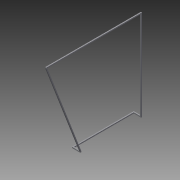
# Autodesk Inventor part: CatchFrameLeft
Saved by Autodesk Inventor 2013 (Build 170138000, 138)
## iProperties
Created: 2014-01-24
Part Number: CatchFrameLeft
Material: Generic
Document SubType Name: Modeling
Designer: Jarod
Density: 1 g/cm^3
Author: Jarod
Autodesk Inventor part; units mm, degrees
ref_plane "YZ Plane" through (0, 0, 0) normal (1, 0, 0) x (0, 1, 0)
ref_plane "XZ Plane" through (0, 0, 0) normal (0, 1, 0) x (-1, 0, 0)
ref_plane "XY Plane" through (0, 0, 0) normal (0, 0, 1) x (1, 0, 0)
sketch "Sketch1" plane through (0, 0, 0) normal (1, 0, 0) x (0, 1, 0)
  line L0 (0, 0) -> (6.35, 0)
  line L1 (6.35, 0) -> (6.35, 381)
  line L2 (6.35, 381) -> (0, 381)
  line L3 (0, 381) -> (0, 0)
  dimension "d0" = 6.35
  dimension "d1" = 381
  constraints: 8 end point, 2 parallel, 1 horizontal, 1 perpendicular
  measures "d0" distance of L2.end L1.end
  measures "d1" distance of L1.end L0.end
extrude "Extrusion1" add sketch "Sketch1" along normal blind 6.35
sketch "Sketch2" plane through (6.35, 0, 0) normal (1, 0, 0) x (0, 0, -1)
  line L0 (-381, 6.35) -> (-374.65, 6.35)
  line L1 (-374.65, 6.35) -> (-374.65, 0)
  line L2 (-374.65, 0) -> (-381, 0)
  line L3 (-381, 0) -> (-381, 6.35)
  line L4 (0, 6.35) -> (-6.35, 6.35)
  line L5 (-6.35, 6.35) -> (-6.35, 0)
  line L6 (-6.35, 0) -> (0, 0)
  line L7 (0, 0) -> (0, 6.35)
  dimension "d4" = 6.35
  dimension "d5" = 6.35
  dimension "d6" = 6.35
  dimension "d7" = 6.35
  constraints: 16 end point, 4 parallel, 2 horizontal, 2 perpendicular
  measures "d4" distance of L1.end L2.end
  measures "d5" distance of L0.end L1.end
  measures "d6" distance of L6.end L5.end
  measures "d7" distance of L5.end L4.end
extrude "Extrusion2" add sketch "Sketch2" along normal blind 38.1
sketch "Sketch3" plane through (44.45, 0, 0) normal (1, 0, 0) x (0, 0, -1)
  line L0 (0, 0) -> (-6.35, 0)
  line L1 (-6.35, 0) -> (-6.35, 558.8)
  line L2 (-6.35, 558.8) -> (0, 558.8)
  line L3 (0, 558.8) -> (0, 0)
  dimension "d10" = 6.35
  dimension "d11" = 558.8
  constraints: 8 end point, 2 parallel, 1 horizontal, 1 perpendicular
  measures "d10" distance of L1.end L2.end
  measures "d11" distance of L0.end L1.end
extrude "Extrusion3" add sketch "Sketch3" along normal blind 6.35
sketch "Sketch4" plane through (50.8, 0, 0) normal (1, 0, 0) x (0, 0, -1)
  line L0 (0, 558.8) -> (-590.55, 558.8)
  line L1 (-590.55, 558.8) -> (-590.55, 552.45)
  line L2 (-590.55, 552.45) -> (0, 552.45)
  line L3 (0, 552.45) -> (0, 558.8)
  dimension "d14" = 590.55
  dimension "d15" = 6.35
  constraints: 8 end point, 2 parallel, 1 horizontal, 1 perpendicular
  measures "d14" distance of L2.end L1.end
  measures "d15" distance of L1.end L0.end
extrude "Extrusion4" add sketch "Sketch4" against normal blind 6.35
sketch "Sketch5" plane through (44.45, 0, 0) normal (1, 0, 0) x (0, 0, -1)
  line L0 (-381, 6.35) -> (-381, 0) projected
  line L1 (-381, 0) -> (-374.65, 0) projected
  line L2 (-374.65, 0) -> (-374.65, 6.35) projected
  line L3 (-374.65, 6.35) -> (-381, 6.35) projected
  line L4 (-381, 6.35) -> (171.45, 6.35) construction
  line L5 (-381, 558.8) -> (-590.55, 558.8)
  line L6 (-590.55, 558.8) -> (-590.55, 552.45)
  line L7 (-590.55, 552.45) -> (-381, 6.35)
  line L8 (-590.55, 558.8) -> (-584.2, 558.8)
  line L9 (-584.2, 558.8) -> (-584.2, 552.45)
  line L10 (-584.2, 552.45) -> (-590.55, 552.45)
  line L11 (-590.55, 552.45) -> (-590.55, 558.8)
  line L12 (-584.2, 552.45) -> (-374.65, 6.35)
  point P0 (0, 0)
  dimension "d18" = 552.45
  dimension "d20" = 209.55
  dimension "d22" = 6.35
  dimension "d23" = 90
  dimension "d24" = 6.35
  dimension "d25" = 6.35
  constraints: 18 end point, 2 horizontal, 2 parallel, 1 perpendicular
  measures "d18" distance of L0.start L5.start
  measures "d20" distance of L5.start L5.end
  measures "d22" distance of L5.end L6.end
  measures "d23" angle of L6 L5
  measures "d24" distance of L9.end L10.end
  measures "d25" distance of L8.end L9.end
extrude "Extrusion5" add sketch "Sketch5" along normal blind 6.35 contours L3 L2 L1 L0 | L7 L10 L12 L3
body "Solid1"
